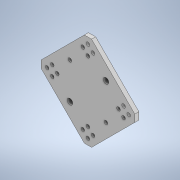
# Autodesk Inventor part: ワイヤジンバル1
Saved by Autodesk Inventor 2020 (Build 240168000, 168)
## iProperties
Created: 2019-10-22
Part Number: ワイヤジンバル1
Material: 一般
Document SubType Name: Modeling
Designer: highs
Density: 1 g/cm^3
Appearance: 既定
Author: highs
## iProperties of the stored document _3D プリント.ipt
Created: 2019-10-23
Part Number: _3D プリント
Material: 一般
Document SubType Name: Modeling
Designer: highs
Density: 1 g/cm^3
Appearance: 既定
Author: highs
Autodesk Inventor part; units mm, degrees
ref_plane "YZ Plane" through (0, 0, 0) normal (1, 0, 0) x (0, 1, 0)
ref_plane "XZ Plane" through (0, 0, 0) normal (0, 1, 0) x (-1, 0, 0)
ref_plane "XY Plane" through (0, 0, 0) normal (0, 0, 1) x (1, 0, 0)
sketch "スケッチ2" plane through (0, 0, 0) normal (0, 0, 1) x (1, 0, 0)
  line L0 (0, -49.4975) -> (49.4975, 0)
  line L1 (49.4975, 0) -> (0, 49.4975)
  line L2 (0, 49.4975) -> (-49.4975, 0)
  line L3 (-49.4975, 0) -> (0, -49.4975)
  line L4 (0, -49.4975) -> (0, 49.4975) construction
  line L5 (49.4975, 0) -> (-49.4975, 0) construction
  circle A0 centre (-5, 35) radius 1.75
  circle A1 centre (5, 35) radius 1.75
  circle A2 centre (-35, -5) radius 1.75
  circle A3 centre (-35, 5) radius 1.75
  circle A4 centre (5, -35) radius 1.75
  circle A5 centre (-5, -35) radius 1.75
  circle A6 centre (35, 5) radius 1.75
  circle A7 centre (35, -5) radius 1.75
  line L6 (-24.7487, 24.7487) -> (24.7487, -24.7487) construction
  line L7 (24.7487, 24.7487) -> (-24.7487, -24.7487) construction
  circle A8 centre (17.6777, 17.6777) radius 2.75
  circle A9 centre (-17.6777, 17.6777) radius 1.75
  circle A10 centre (-17.6777, -17.6777) radius 2.75
  circle A11 centre (17.6777, -17.6777) radius 1.75
  circle A12 centre (-30, 0) radius 1.75
  circle A13 centre (-40, 0) radius 1.75
  line L8 (-35, -5) -> (-35, 5) construction
  circle A14 centre (0, -30) radius 1.75
  circle A15 centre (0, -40) radius 1.75
  circle A16 centre (30, 0) radius 1.75
  circle A17 centre (40, 0) radius 1.75
  circle A18 centre (0, 30) radius 1.75
  circle A19 centre (0, 40) radius 1.75
  point P0 (0, 0)
  dimension "d1" = 3.5
  dimension "d2" = 5
  dimension "d3" = 35
  dimension "d6" = 360
  dimension "d12" = 5.5
  dimension "d13" = 3.5
  dimension "d14" = 25
  dimension "d15" = 25
  dimension "d29" = 70
  dimension "d30" = 5
  dimension "d31" = 5
  dimension "d34" = 360
  constraints: 20 centre point, 18 end point, 6 midpoint, 4 point on line, 3 symmetric about line, 2 equal radius, 2 parallel, 2 perpendicular, 1 horizontal, 1 vertical, 37 other
  measures "d1" diameter of A0
  measures "d2" distance from line of L4 A0.centre
  measures "d3" distance from line of L5 A0.centre
  measures "d12" diameter of A8
  measures "d13" diameter of A9
  measures "d14" distance from line of L6 A8.centre
  measures "d15" distance from line of L7 A9.centre
  measures "d29" distance between parallel lines of L3 L1
  measures "d30" distance from line of A12.centre L8
  measures "d31" distance from line of L8 A13.centre
extrude "押し出し1" add sketch "スケッチ2" along normal blind 4
chamfer "面取り1" distance 5 angle 45 4 edges at (0, -49.4975, 2) (49.4975, 0, 2) (0, 49.4975, 2) (-49.4975, 0, 2)
